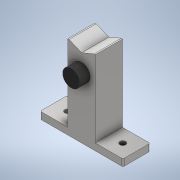
# Autodesk Inventor part: Stop sliding
Saved by Autodesk Inventor 2021 (Build 250183000, 183)
## iProperties
Created: 2021-06-07
Part Number: Stop sliding
Material: Generic
Document SubType Name: Modeling
Designer: Nelson
Density: 1 g/cm^3
Appearance: Default
Author: Nelson
Autodesk Inventor part; units mm, degrees
ref_plane "YZ Plane" through (0, 0, 0) normal (1, 0, 0) x (0, 1, 0)
ref_plane "XZ Plane" through (0, 0, 0) normal (0, 1, 0) x (-1, 0, 0)
ref_plane "XY Plane" through (0, 0, 0) normal (0, 0, 1) x (1, 0, 0)
sketch "Sketch3" plane through (0, 0, 0) normal (0, 0, 1) x (1, 0, 0)
  line L0 (0, 0) -> (60, 0)
  line L1 (60, 0) -> (60, 10)
  line L2 (60, 10) -> (20, 10)
  line L3 (20, 10) -> (20, 120.986)
  line L4 (0, 0) -> (0, 29.8306) construction
  line L5 (0, 0) -> (-60, 0)
  line L6 (-60, 0) -> (-60, 10)
  line L7 (-60, 10) -> (-20, 10)
  line L8 (-20, 10) -> (-20, 120.986)
  line L9 (799.716, 113.486) -> (799.716, 376.2074) construction
  line L10 (0, 113.486) -> (18.1144, 120.986)
  line L11 (18.1144, 120.986) -> (20, 120.986)
  line L12 (-18.1144, 120.986) -> (0, 113.486)
  line L13 (-20, 120.986) -> (-18.1144, 120.986)
  dimension "d10" = 60
  dimension "d11" = 10
  dimension "d41" = 18.1144
  dimension "d44" = 110.986
  dimension "d45" = 7.5
  dimension "d46" = 40
  dimension "d47" = 110.986
  constraints: 28 end point, 4 horizontal, 3 symmetric about line, 3 vertical, 1 equal length, 1 perpendicular
  measures "d10" distance of L0.start L0.end
  measures "d11" distance of L0.end L1.end
  measures "d41" horizontal distance of L12.end L12.start
  measures "d44" distance of L8.start L8.end
  measures "d45" distance from line of L12.end L13
  measures "d46" distance of L7.start L8.start
  measures "d47" distance of L3.end L2.end
extrude "Extrusion1" add sketch "Sketch3" against normal blind 39.3
sketch "Sketch4" plane through (0, 0, 0) normal (0, 0, 1) x (1, 0, 0)
  circle A0 centre (0, 89) radius 12.5
  point P0 (0, 0)
  dimension "d20" = 25
  constraints: 1 centre point, 1 coincident
  measures "d20" diameter of A0
extrude "Extrusion2" add sketch "Sketch4" along normal blind 15
fillet "Fillet1" radius 2 4 edges at (60, 5, 0) (60, 5, -39.3) (-60, 5, 0) (-60, 5, -39.3)
sketch "Sketch5" plane through (-20, 10, 0) normal (0, 1, 0) x (1, 0, 0)
  line L0 (-38, 39.3) -> (0, 39.3) projected
  line L1 (40, 39.3) -> (78, 39.3) projected
  line L2 (-40, 2) -> (-40, 37.3) projected
  line L3 (80, 2) -> (80, 37.3) projected
  point P0 (20, 0)
  point P1 (-20, 19.65)
  point P2 (60, 19.65)
  dimension "d24" = 19.65
  dimension "d25" = 19.65
  dimension "d26" = 20
  dimension "d27" = 20
  measures "d24" distance from line of point (-20, 19.65) L0
  measures "d25" distance from line of L1 point (60, 19.65)
  measures "d26" distance from line of point (-20, 19.65) L2
  measures "d27" distance from line of point (60, 19.65) L3
hole "Hole1" at (-40, 10, -19.65) at (40, 10, -19.65) direction (0, -1, 0) diameter 8.376 end through all thread size "M10x1.5" class "6H" standard "ISO Metric profile"
equation "\"d47\" = d44"
equation "\"d25\" = d24"
equation "\"d27\" = d26"
body "Solid1"
